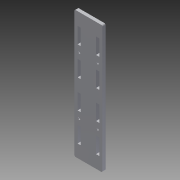
# Autodesk Inventor part: BatPlate
Saved by Autodesk Inventor 2015 (Build 190159000, 159)
## iProperties
Created: 2016-03-02
Part Number: BatPlate
Material: ABS Plastic
Document SubType Name: Modeling
Designer: Eric
Density: 1.06 g/cm^3
Appearance: Smooth - White
Mass: 41.1513 g
Surface Area: 205.527 cm^2
Volume: 38.822 cm^3
Author: Eric
Autodesk Inventor part; units mm, degrees
ref_plane "YZ Plane" through (0, 0, 0) normal (1, 0, 0) x (0, 1, 0)
sketch "Sketch1" plane through (0, 0, 0) normal (0, 1, 0) x (-1, 0, 0)
  line L0 (0, 0) -> (0, -200)
  line L1 (0, -200) -> (44, -200)
  line L2 (44, -200) -> (44, 0)
  line L3 (44, 0) -> (0, 0)
  dimension "d0" = 200
  dimension "d1" = 44
  constraints: 8 end point, 3 perpendicular, 1 vertical
  measures "d0" distance of L0.start L0.end
  measures "d1" distance of L0.end L1.end
extrude "Extrusion1" add sketch "Sketch1" along normal blind 5
sketch "Sketch2" plane through (0, 5, 0) normal (0, 1, 0) x (1, 0, 0)
  line L0 (-10, 8) -> (-10, 208)
  line L1 (-10, 208) -> (-30, 208)
  line L2 (-30, 208) -> (-30, 8)
  line L3 (-30, 8) -> (-10, 8)
  line L4 (-10, 8) -> (-30, 208) construction
  line L5 (-10, 208) -> (-30, 8) construction
  line L6 (0, 200) -> (-44, 200) projected
  line L7 (-44, 0) -> (0, 0) projected
  line L8 (0, 0) -> (0, 200) projected
  line L9 (-35, 0) -> (-35, 200)
  line L10 (-5, 0) -> (-5, 200)
  line L11 (-35, 10) -> (-30, 10)
  line L12 (-10, 20) -> (-5, 20)
  line L13 (-35, 35) -> (-30, 35)
  line L14 (-10, 45) -> (-5, 45)
  line L15 (-35, 55) -> (-30, 55)
  line L16 (-10, 65) -> (-5, 65)
  line L17 (-35, 80) -> (-30, 80)
  line L18 (-10, 90) -> (-5, 90)
  point P0 (-20, 108)
  dimension "d4" = 200
  dimension "d5" = 20
  dimension "d6" = 108
  dimension "d8" = 5
  dimension "d9" = 5
  dimension "d14" = 10
  dimension "d15" = 25
  dimension "d16" = 20
  dimension "d17" = 25
  dimension "d18" = 20
  dimension "d19" = 25
  dimension "d20" = 20
  dimension "d21" = 25
  dimension "d41" = 5
  constraints: 32 end point, 20 point on line, 12 perpendicular, 2 midpoint, 2 parallel
  measures "d4" distance of L0.start L0.end
  measures "d5" distance of L1.end L0.end
  measures "d6" distance from line of point (-20, 108) L7
  measures "d8" distance between parallel lines of L2 L9
  measures "d9" distance between parallel lines of L0 L10
  measures "d14" distance between parallel lines of L7 L11
  measures "d15" distance between parallel lines of L11 L13
  measures "d16" distance between parallel lines of L13 L15
  measures "d17" distance between parallel lines of L15 L17
  measures "d18" distance between parallel lines of L7 L12
  measures "d19" distance between parallel lines of L12 L14
  measures "d20" distance between parallel lines of L14 L16
  measures "d21" distance between parallel lines of L16 L18
  measures "d41" distance between parallel lines of L8 L10
extrude "Extrusion2" cut sketch "Sketch2" against normal blind 5 contours L0 L14 L10 L12 | L0 L18 L10 L16
ref_plane "Work Plane1" through (-22, 0, 0) normal (1, 0, 0) x (0, 0, -1)
ref_plane "Work Plane2" through (0, 0, -100) normal (0, 0, -1) x (-1, 0, 0)
mirror "Mirror1" about plane through (-22, 0, 0) normal (1, 0, 0) of "Extrusion2"
mirror "Mirror2" about plane through (0, 0, -100) normal (0, 0, -1) of "Extrusion2", "Mirror1"
sketch "Sketch5" plane through (0, 5, 0) normal (0, 1, 0) x (1, 0, 0)
  circle A0 centre (-7.5, 55) radius 1.6
  line L0 (-10, 45) -> (-5, 45) projected
  line L1 (-5, 45) -> (-5, 20) projected
  line L2 (0, 0) -> (0, 200) projected
  line L3 (0, 100) -> (-44, 100)
  line L4 (-44, 200) -> (-44, 0) projected
  line L5 (0, 200) -> (-44, 200) projected
  line L6 (-22, 200) -> (-22, 0)
  line L7 (-44, 0) -> (0, 0) projected
  circle A1 centre (-7.5, 145) radius 1.6
  circle A2 centre (-36.5, 55) radius 1.6
  circle A3 centre (-36.5, 145) radius 1.6
  dimension "d42" = 3.2
  dimension "d43" = 10
  dimension "d44" = 2.5
  constraints: 4 centre point, 4 end point, 4 midpoint, 3 symmetric about line, 3 other
  measures "d42" diameter of A0
  measures "d43" distance from line of L0 A0.centre
  measures "d44" distance from line of A0.centre L1
extrude "Extrusion4" cut sketch "Sketch5" against normal blind 5 contours A0 | A1 | A2 | A3
fillet "Fillet1" radius 2 4 edges at (-44, 2.5, 0) (0, 2.5, 0) (0, 2.5, -200) (-44, 2.5, -200)
body "Solid1"
